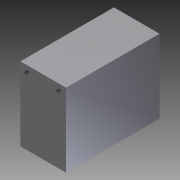
# Autodesk Inventor part: Y axis home sensor block
Saved by Autodesk Inventor 2011 (Build 150239000, 239)
## iProperties
Created: 2014-04-04
Part Number: Y axis home sensor block
Document SubType Name: Modeling
Designer: Devon
Density: 1 g/cm^3
Author: Devon
Autodesk Inventor part; units mm, degrees
ref_plane "YZ Plane" through (0, 0, 0) normal (1, 0, 0) x (0, 1, 0)
ref_plane "XZ Plane" through (0, 0, 0) normal (0, 1, 0) x (-1, 0, 0)
ref_plane "XY Plane" through (0, 0, 0) normal (0, 0, 1) x (1, 0, 0)
sketch "Sketch1" plane through (0, 0, 0) normal (0, 0, 1) x (1, 0, 0)
  line L0 (-15.8425, 1.2211) -> (3.8425, 1.2211)
  line L1 (3.8425, 1.2211) -> (3.8425, -30.5035)
  line L2 (3.8425, -30.5035) -> (-15.8425, -30.5035)
  line L3 (-15.8425, -30.5035) -> (-15.8425, 1.2211)
  point P0 (0, 0)
  dimension "d0" = 19.685
  dimension "d1" = 31.7246
  constraints: 8 end point, 2 parallel, 1 horizontal, 1 perpendicular
  measures "d0" distance of L1.end L2.end
  measures "d1" distance of L0.end L1.end
extrude "Extrusion1" add sketch "Sketch1" along normal blind 40.3352
sketch "Sketch3" plane through (0, 0, 40.3352) normal (0, 0, 1) x (1, 0, 0)
  line L0 (-15.8425, 1.2211) -> (3.8425, 1.2211) projected
  line L1 (-15.8425, 1.2211) -> (-12.8453, 1.2211)
  line L2 (-12.8453, 1.2211) -> (-12.8453, -1.7761)
  line L3 (3.8425, 1.2211) -> (0.8453, 1.2211)
  line L4 (0.8453, 1.2211) -> (0.8453, -1.7761)
  point P0 (0, 0)
  dimension "d4" = 2.9972
  dimension "d5" = 2.9972
  dimension "d6" = 2.9972
  constraints: 8 end point, 2 perpendicular, 2 point on line
  measures "d4" distance of L0.start L1.end
  measures "d5" distance of L1.end L2.end
  measures "d6" distance of L0.end L3.end
hole "Hole1" at (-12.8453, -1.7761, 40.3352) at (0.8453, -1.7761, 40.3352) direction (0, 0, -1) diameter 2.4892 depth 12.7 tip angle 118
body "Solid1"
